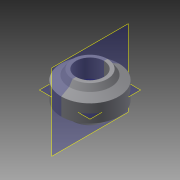
# Autodesk Inventor part: Spacer
Saved by Autodesk Inventor 2018.2 (Build 222227000, 227)
## iProperties
Created: 2018-02-28
Part Number: Spacer
Material: Generic
Document SubType Name: Modeling
Designer: Rus
Density: 1 g/cm^3
Appearance: Default
Author: Rus
Autodesk Inventor part; units mm, degrees
ref_plane "YZ Plane" through (0, 0, 0) normal (1, 0, 0) x (0, 1, 0)
sketch "Sketch1" plane through (0, 0, 0) normal (0, 0, 1) x (1, 0, 0)
  circle A0 centre (0, 0) radius 4
  circle A1 centre (0, 0) radius 6
  line L0 (0, 0) -> (0, 6) construction
  line L1 (0, 0) -> (-6, 0) construction
  dimension "d0" = 8
  dimension "d1" = 12
  constraints: 4 end point, 2 centre point, 2 coincident, 2 point on circle, 1 perpendicular, 1 vertical
  measures "d0" diameter of A0
  measures "d1" diameter of A1
ref_plane "Work Plane1" through (0, 0, 0) normal (0, 0, -1) x (-1, 0, 0)
ref_plane "Work Plane2" through (-9, -9, -5.25) normal (0, 0, -1) x (0, 1, 0)
ref_plane "Work Plane3" through (-9, -9, 5.25) normal (0, 0, 1) x (1, 0, 0)
extrude "Extrusion1" add sketch "Sketch1" along normal up to surface (10.5 mm away) from surface at -5.25
chamfer "Chamfer1" distance 1.5 distance2 1 1 edges at (-6, 0, -5.25) measured on face at (-6, 0, -4.75)
chamfer "Chamfer2" distance 1.5 distance2 1 1 edges at (-6, 0, 5.25) measured on face at (-6, 0, 4.75)
ref_plane "Work Plane4" through (0, 0, 0) normal (-1, 0, 0) x (0, -1, 0)
sketch "Sketch2" plane through (0, 0, 0) normal (-1, 0, 0) x (0, -1, 0)
  line L0 (-6, -3.75) -> (-6, 3.75) construction
  line L1 (-5, -5.25) -> (-6, -3.75) construction
  line L2 (-4, -5.25) -> (-4, 5.25) construction
  line L3 (9, 5.25) -> (-9, 5.25) construction
  line L4 (-5, 5.25) -> (-6, 3.75) construction
  line L5 (-8.25, -2.5) -> (-8.25, 2.5)
  line L6 (-9, -5.25) -> (-9, 5.25) construction
  line L7 (-6, 0) -> (-8.25, 0) construction
  line L8 (-6, -3.75) -> (-6, 3.75)
  line L9 (-4, -5.25) -> (4, -5.25) projected
  line L10 (0, -5.25) -> (0, 5.25)
  line L11 (-8.25, -2.5) -> (-6, -3.75)
  line L12 (-6, 3.75) -> (-8.25, 2.5)
  point P0 (0, 0)
  dimension "d10" = 5
  dimension "d12" = 0.75
  constraints: 16 end point, 4 midpoint, 2 vertical, 1 collinear, 1 horizontal, 3 other
  measures "d10" distance of L5.start L5.end
  measures "d12" distance between parallel lines of L6 L5
revolve "Revolution1" add sketch "Sketch2" angle 360 about axis through (0, 0, -5.25) along (0, 0, 1)
body "Solid1"
